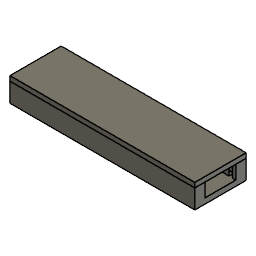
LD2410B Mount v3 (Autodesk Fusion 360 design; units mm, degrees)
Autodesk Fusion 360 part; units mm, degrees
sketch "Sketch1" plane through (0, 0, 0) normal (0, 1, 0) x (1, 0, 0)
  line L0 (23, -3.5) -> (-23, -3.5)
  line L1 (-23, -3.5) -> (-23, 3.5)
  line L2 (-23, 3.5) -> (23, 3.5)
  line L3 (23, 3.5) -> (23, -3.5)
  line L4 (23, -3.5) -> (-23, 3.5) construction
  line L5 (-23, -3.5) -> (23, 3.5) construction
  line L6 (24, -4.5) -> (-24, -4.5)
  line L7 (-24, -4.5) -> (-24, 4.5)
  line L8 (-24, 4.5) -> (24, 4.5)
  line L9 (24, 4.5) -> (24, -4.5)
  line L10 (25, -5.5) -> (-25, -5.5)
  line L11 (-25, -5.5) -> (-25, 5.5)
  line L12 (-25, 5.5) -> (25, 5.5)
  line L13 (25, 5.5) -> (25, -5.5)
  line L14 (26, -6.5) -> (-26, -6.5)
  line L15 (-26, -6.5) -> (-26, 6.5)
  line L16 (-26, 6.5) -> (26, 6.5)
  line L17 (26, 6.5) -> (26, -6.5)
  line L18 (27, -7.5) -> (-27, -7.5)
  line L19 (-27, -7.5) -> (-27, 7.5)
  line L20 (-27, 7.5) -> (27, 7.5)
  line L21 (27, 7.5) -> (27, -7.5)
  line L22 (9, 4.5) -> (9, -4.5)
  line L23 (24, 4.5) -> (27, 4.5)
  line L24 (24, -4.5) -> (27, -4.5)
  dimension "d1" = 46
  dimension "d2" = 7
  dimension "d3" = -1
  dimension "d4" = -1
  dimension "d5" = -1
  dimension "d6" = -1
  dimension "d7" = 32
  constraint horizontal L0
  constraint perpendicular L0 L1
  constraint parallel L0 L2
  constraint parallel L1 L3
  constraint coincident L4 origin
  constraint coincident L5 origin
  constraint coincident L8 L22.start
  constraint coincident L6 L22.end
  constraint perpendicular L6 L22
  constraint coincident L21 L23.end
  constraint perpendicular L21 L23
  constraint coincident L21 L24.end
  constraint perpendicular L21 L24
  measures "d1" distance of L1.end L2.end
  measures "d2" distance of L0.end L1.end
  measures "d7" distance of L1 L22
extrude "Extrude1" add sketch "Sketch1" along normal blind 1.6 contours L0 L2 L3 L6 L8 L9 L22 | L0 L2 L3 L22 | L0 L1 L2 L22 | L9 L13 L23 L24 | L10 L11 L12 L13 L14 L15 L16 L17 L23 L24 | L13 L17 L23 L24 | L17 L21 L23 L24 makes body 1
extrude "Extrude2" add sketch "Sketch1" along normal blind 5.6 contours L0 L1 L2 L6 L7 L8 L22 | L6 L7 L8 L10 L11 L12 L13 L23 L24 | L14 L15 L16 L17 L18 L19 L20 L21 L23 L24 bodies 1
move_body "Move1" bodies 1 to x (1, 0, 0) y (0, 1, 0) z (0, 0, 1) at (0, 0, -32.7089)
sketch "Sketch2" plane through (0, 0, 0) normal (0, 1, 0) x (1, 0, 0)
  line L0 (27, -7.5) -> (-27, -7.5)
  line L1 (-27, -7.5) -> (-27, 7.5)
  line L2 (-27, 7.5) -> (27, 7.5)
  line L3 (27, 7.5) -> (27, -7.5)
  line L4 (27, -7.5) -> (-27, 7.5) construction
  line L5 (-27, -7.5) -> (27, 7.5) construction
  line L6 (25.975, -6.475) -> (-25.975, -6.475)
  line L7 (-25.975, -6.475) -> (-25.975, 6.475)
  line L8 (-25.975, 6.475) -> (25.975, 6.475)
  line L9 (25.975, 6.475) -> (25.975, -6.475)
  line L10 (25.975, -6.475) -> (-25.975, 6.475) construction
  line L11 (-25.975, -6.475) -> (25.975, 6.475) construction
  line L12 (25.025, -5.525) -> (-25.025, -5.525)
  line L13 (-25.025, -5.525) -> (-25.025, 5.525)
  line L14 (-25.025, 5.525) -> (25.025, 5.525)
  line L15 (25.025, 5.525) -> (25.025, -5.525)
  line L16 (25.025, -5.525) -> (-25.025, 5.525) construction
  line L17 (-25.025, -5.525) -> (25.025, 5.525) construction
  line L18 (25.025, 4.5) -> (27, 4.5)
  line L19 (25.025, -4.5) -> (27, -4.5)
  dimension "d29" = 54
  dimension "d30" = 15
  dimension "d31" = 51.95
  dimension "d32" = 12.95
  dimension "d33" = 11.05
  dimension "d34" = 50.05
  dimension "d35" = 3
  dimension "d36" = 3
  constraint horizontal L0
  constraint perpendicular L0 L1
  constraint parallel L0 L2
  constraint parallel L1 L3
  constraint coincident L4 origin
  constraint coincident L5 origin
  constraint horizontal L6
  constraint perpendicular L6 L7
  constraint parallel L6 L8
  constraint parallel L7 L9
  constraint coincident L10 origin
  constraint coincident L11 origin
  constraint horizontal L12
  constraint perpendicular L12 L13
  constraint parallel L12 L14
  constraint parallel L13 L15
  constraint coincident L16 origin
  constraint coincident L17 origin
  constraint coincident L15 L18.start
  constraint coincident L3 L18.end
  constraint perpendicular L3 L18
  constraint coincident L15 L19.start
  constraint coincident L3 L19.end
  constraint perpendicular L3 L19
  measures "d29" distance of L1.end L2.end
  measures "d30" distance of L0.end L1.end
  measures "d31" distance of L7.end L8.end
  measures "d32" distance of L6.end L7.end
  measures "d33" distance of L12 L14
  measures "d34" distance of L13 L15
  measures "d35" distance of L0 L19
  measures "d36" distance of L2 L18
extrude "Extrude7" add sketch "Sketch2" along normal blind 1.4 separate body contours L0 L1 L2 L3 L6 L7 L8 L9 L18 L19 | L3 L9 L18 L19 | L9 L15 L18 L19 | L12 L13 L14 L15 makes body 2
extrude "Extrude8" add sketch "Sketch2" along normal blind 4 contours L6 L7 L8 L9 L12 L13 L14 L15 L18 L19 bodies 2
copy_body "Body->Comp1" bodies 1 removing the originals makes body 3 in component "LD2410B_Mount_Body"
copy_body "Body->Comp3" bodies 2 removing the originals makes body 4 in component "LD2410B_Mount_Top"
component "LD2410B_Mount_Body" placed x (1, 0, 0) y (0, 1, 0) z (0, 0, 1) at (0, 0, 0)
component "LD2410B_Mount_Top" placed x (1, 0, 0) y (0, -1, 0) z (0, 0, -1) at (0, 7, -32.7089)
